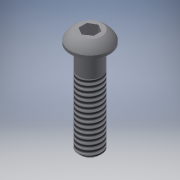
# Autodesk Inventor part: Caufield_Axle_Peg
Saved by Autodesk Inventor 2016 (Build 200138000, 138)
## iProperties
Created: 2018-01-10
Part Number: Caufield_Axle_Peg
Material: Generic
Document SubType Name: Modeling
Designer: caufield58738
Density: 1 g/cm^3
Appearance: Default
Mass: 0.984327 g
Surface Area: 7.74345 cm^2
Volume: 0.984327 cm^3
Author: caufield58738
Autodesk Inventor part; units mm, degrees
ref_plane "YZ Plane" through (0, 0, 0) normal (1, 0, 0) x (0, 1, 0)
ref_plane "XZ Plane" through (0, 0, 0) normal (0, 1, 0) x (-1, 0, 0)
ref_plane "XY Plane" through (0, 0, 0) normal (0, 0, 1) x (1, 0, 0)
sketch "Bolt sketch" plane through (0, 0, 0) normal (0, 0, 1) x (1, 0, 0)
  circle A0 centre (0, 0) radius 3.175
  dimension "d0" = 6.35
  constraints: 1 centre point, 1 coincident
  measures "d0" diameter of A0
extrude "Bolt extrution" add sketch "Bolt sketch" along normal blind 25.4
thread "Axle peg Thread" size "1/4-20 UNC" class "2A" standard "ANSI Unified Screw Threads" length 19.05 offset 6.35
sketch "Head Sketch" plane through (0, 0, 0) normal (1, 0, 0) x (0, 1, 0)
  line L0 (3.175, 25.4) -> (-3.175, 25.4) projected
  line L1 (0, 25.4) -> (5.3594, 25.4)
  line L2 (5.3594, 25.4) -> (5.3594, 26.1874)
  line L3 (0, 25.4) -> (0, 28.575)
  line L4 (0, 28.575) -> (3.175, 28.575)
  arc A0 (5.3594, 26.1874) -> (3.175, 28.575) centre (0.0087, 23.4851) ccw
  point P0 (0, 0)
  dimension "d5" = 5.3594
  dimension "d6" = 0.7874
  dimension "d7" = 3.175
  dimension "d8" = 3.175
  dimension "d9" = 5.9944
  constraints: 8 end point, 2 horizontal, 2 point on circle, 1 centre point, 1 midpoint, 1 perpendicular, 1 vertical
  measures "d5" distance of L1.start L1.end
  measures "d6" distance of L1.end L2.end
  measures "d7" distance of L1.start L3.end
  measures "d8" distance of L3.end L4.end
  measures "d9" radius of A0
revolve "Revolution1" add sketch "Head Sketch" angle 360 about axis through (0, 0, 25.4) along (0, 0, 1)
sketch "Hexagon sketch" plane through (0, 0, 28.575) normal (0, 0, 1) x (1, 0, 0)
  line L0 (1.1498, -1.9844) -> (-1.1498, -1.9844)
  line L1 (-1.1498, -1.9844) -> (-2.2873, 0)
  line L2 (-2.2873, 0) -> (-1.1498, 1.9844)
  line L3 (-1.1498, 1.9844) -> (1.1569, 1.9844)
  line L4 (1.1569, 1.9844) -> (2.2873, 0)
  line L5 (2.2873, 0) -> (1.1498, -1.9844)
  line L6 (0, 0) -> (3.4356, 0) construction
  line L7 (0, 0) -> (-2.586, 0) construction
  dimension "d13" = 3.9688
  dimension "d15" = 3.9688
  dimension "d16" = 0.156
  dimension "d17" = 1.9844
  dimension "d18" = 1.9844
  dimension "d19" = 1.9844
  dimension "d20" = 1.9875
  constraints: 16 end point, 2 horizontal, 2 parallel, 2 point on line
  measures "d13" distance between parallel lines of L5 L2
  measures "d15" distance between parallel lines of L0 L3
  measures "d16" angle of L1 L4
  measures "d17" distance from line of L0 L6.start
  measures "d18" distance from line of L6.start L1
  measures "d19" distance from line of L2 L6.start
  measures "d20" distance from line of L4 L6.start
extrude "Hexagon Hole extrution" cut sketch "Hexagon sketch" against normal blind 2.8194
chamfer "Bottom Chamfer" distance 0.762 angle 45 1 edges at (-3.175, 0, 0)
body "Solid1"
